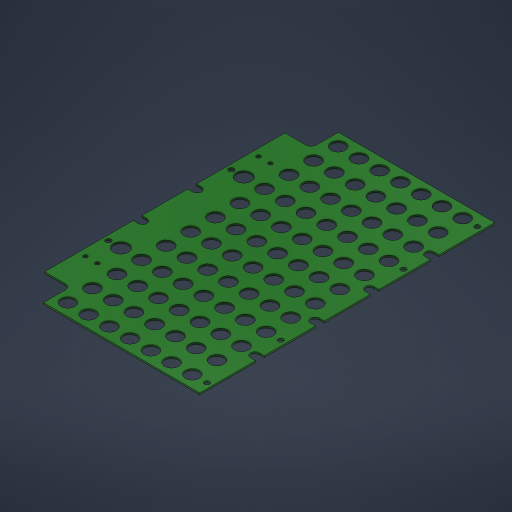
# Autodesk Inventor part: PCB
Saved by Autodesk Inventor 2023.5 (Build 275446000, 446)
## iProperties
Created: 2025-03-26
Part Number: PCB
Material: PC/ABS-Kunststoff
Document SubType Name: Modeling
Designer: David Lill
Density: 0.357273 g/cm^3
Appearance: Glatt - Waldgrün
Author: David Lill
Autodesk Inventor part; units mm, degrees
ref_plane "YZ Plane" through (0, 0, 0) normal (1, 0, 0) x (0, 1, 0)
ref_plane "XZ Plane" through (0, 0, 0) normal (0, 1, 0) x (-1, 0, 0)
ref_plane "XY Plane" through (0, 0, 0) normal (0, 0, 1) x (1, 0, 0)
sketch "Skizze1" plane through (0, 0, 0) normal (0, 0, 1) x (1, 0, 0)
  arc A0 (0, 11.25) -> (-14.9586, 20.25) centre (-14.9586, 3.3189) ccw
  arc A1 (-14.9586, 2.25) -> (-14.9586, 20.25) centre (-18, 11.25) ccw
  arc A2 (-14.9586, 2.25) -> (0, 11.25) centre (-14.9586, 19.1811) ccw
  arc A3 (0, 78.75) -> (-14.9586, 87.75) centre (-14.9586, 70.8189) ccw
  arc A4 (-14.9586, 69.75) -> (-14.9586, 87.75) centre (-18, 78.75) ccw
  arc A5 (-14.9586, 69.75) -> (0, 78.75) centre (-14.9586, 86.6811) ccw
  line L0 (0, 0) -> (0, 270)
  arc A6 (-4.65, 164) -> (-4.65, 156) centre (-4.65, 160) ccw
  line L1 (-4.65, 156) -> (0, 156)
  line L2 (0, 0) -> (0, 270)
  arc A7 (-4.65, 219) -> (-4.65, 211) centre (-4.65, 215) ccw
  line L3 (-4.65, 211) -> (0, 211)
  line L4 (0, 135) -> (-167, 135)
  line L5 (0, 270) -> (-167, 270)
  line L6 (-167, 270) -> (-167, 0)
  line L7 (-167, 270) -> (-167, 0)
  line L8 (-167, 0) -> (0, 0)
  line L9 (0, 0) -> (-167, 0)
  line L10 (-144.5, 31.5) -> (-165.5, 31.5)
  line L11 (-165.5, 31.5) -> (-165.5, 58.5)
  line L12 (-165.5, 58.5) -> (-144.5, 58.5)
  line L13 (-144.5, 58.5) -> (-144.5, 31.5)
  line L14 (-144.5, 238.5) -> (-165.5, 238.5)
  line L15 (-165.5, 238.5) -> (-165.5, 211.5)
  line L16 (-165.5, 211.5) -> (-144.5, 211.5)
  line L17 (-144.5, 211.5) -> (-144.5, 238.5)
  arc A8 (0, 258.75) -> (-14.9586, 267.75) centre (-14.9586, 250.8189) ccw
  arc A9 (-14.9586, 249.75) -> (0, 258.75) centre (-14.9586, 266.6811) ccw
  arc A10 (-14.9586, 249.75) -> (-14.9586, 267.75) centre (-18, 258.75) ccw
  arc A11 (0, 191.25) -> (-14.9586, 200.25) centre (-14.9586, 183.3189) ccw
  arc A12 (-14.9586, 182.25) -> (-14.9586, 200.25) centre (-18, 191.25) ccw
  arc A13 (-14.9586, 182.25) -> (0, 191.25) centre (-14.9586, 199.1811) ccw
  line L18 (-135.0414, 87.75) -> (-158, 87.75)
  arc A14 (-158, 87.75) -> (-158, 69.75) centre (-158, 78.75) ccw
  line L19 (-158, 69.75) -> (-135.0414, 69.75)
  arc A15 (-135.0414, 87.75) -> (-135.0414, 69.75) centre (-132, 78.75) ccw
  line L20 (-158, 182.25) -> (-135.0414, 182.25)
  arc A16 (-135.0414, 200.25) -> (-135.0414, 182.25) centre (-132, 191.25) ccw
  line L21 (-135.0414, 200.25) -> (-158, 200.25)
  arc A17 (-158, 200.25) -> (-158, 182.25) centre (-158, 191.25) ccw
  line L22 (-143, 0) -> (-143, 55)
  arc A18 (-143, 55) -> (-148, 60) centre (-148, 55) ccw
  line L23 (-148, 60) -> (-167, 60)
  line L24 (-167, 25) -> (-148, 25)
  arc A19 (-143, 20) -> (-148, 25) centre (-148, 20) ccw
  line L25 (-143, 270) -> (-143, 215)
  arc A20 (-148, 210) -> (-143, 215) centre (-148, 215) ccw
  line L26 (-148, 210) -> (-167, 210)
  line L27 (-167, 245) -> (-148, 245)
  arc A21 (-148, 245) -> (-143, 250) centre (-148, 250) ccw
  line L28 (0, 219) -> (-4.65, 219)
  arc A22 (-4.65, 219) -> (-4.65, 211) centre (-4.65, 215) ccw
  line L29 (-4.65, 211) -> (0, 211)
  line L30 (0, 164) -> (-4.65, 164)
  arc A23 (-4.65, 164) -> (-4.65, 156) centre (-4.65, 160) ccw
  line L31 (-4.65, 156) -> (0, 156)
  line L32 (-167, 156) -> (-162.35, 156)
  arc A24 (-162.35, 156) -> (-162.35, 164) centre (-162.35, 160) ccw
  line L33 (-162.35, 164) -> (-167, 164)
  line L34 (0, 59) -> (-4.65, 59)
  arc A25 (-4.65, 59) -> (-4.65, 51) centre (-4.65, 55) ccw
  line L35 (-4.65, 51) -> (0, 51)
  line L36 (0, 106) -> (-4.65, 106)
  arc A26 (-4.65, 114) -> (-4.65, 106) centre (-4.65, 110) ccw
  line L37 (-4.65, 114) -> (0, 114)
  line L38 (-167, 106) -> (-162.35, 106)
  arc A27 (-162.35, 106) -> (-162.35, 114) centre (-162.35, 110) ccw
  line L39 (-162.35, 114) -> (-167, 114)
  circle A28 centre (-18, 236.25) radius 9
  circle A29 centre (-18, 258.75) radius 9
  circle A30 centre (-18, 213.75) radius 9
  circle A31 centre (-18, 168.75) radius 9
  circle A32 centre (-18, 123.75) radius 9
  circle A33 centre (-18, 78.75) radius 9
  circle A34 centre (-18, 33.75) radius 9
  circle A35 centre (-18, 11.25) radius 9
  circle A36 centre (-18, 56.25) radius 9
  circle A37 centre (-18, 101.25) radius 9
  circle A38 centre (-18, 146.25) radius 9
  circle A39 centre (-18, 191.25) radius 9
  circle A40 centre (-37, 236.25) radius 9
  circle A41 centre (-37, 258.75) radius 9
  circle A42 centre (-37, 213.75) radius 9
  circle A43 centre (-37, 168.75) radius 9
  circle A44 centre (-37, 123.75) radius 9
  circle A45 centre (-37, 78.75) radius 9
  circle A46 centre (-37, 33.75) radius 9
  circle A47 centre (-37, 11.25) radius 9
  circle A48 centre (-37, 56.25) radius 9
  circle A49 centre (-37, 101.25) radius 9
  circle A50 centre (-37, 146.25) radius 9
  circle A51 centre (-37, 191.25) radius 9
  circle A52 centre (-56, 236.25) radius 9
  circle A53 centre (-56, 258.75) radius 9
  circle A54 centre (-56, 213.75) radius 9
  circle A55 centre (-56, 168.75) radius 9
  circle A56 centre (-56, 123.75) radius 9
  circle A57 centre (-56, 78.75) radius 9
  circle A58 centre (-56, 33.75) radius 9
  circle A59 centre (-56, 11.25) radius 9
  circle A60 centre (-56, 56.25) radius 9
  circle A61 centre (-56, 101.25) radius 9
  circle A62 centre (-56, 146.25) radius 9
  circle A63 centre (-56, 191.25) radius 9
  circle A64 centre (-75, 236.25) radius 9
  circle A65 centre (-75, 258.75) radius 9
  circle A66 centre (-75, 213.75) radius 9
  circle A67 centre (-75, 168.75) radius 9
  circle A68 centre (-75, 123.75) radius 9
  circle A69 centre (-75, 78.75) radius 9
  circle A70 centre (-75, 33.75) radius 9
  circle A71 centre (-75, 11.25) radius 9
  circle A72 centre (-75, 56.25) radius 9
  circle A73 centre (-75, 101.25) radius 9
  circle A74 centre (-75, 146.25) radius 9
  circle A75 centre (-75, 191.25) radius 9
  circle A76 centre (-94, 236.25) radius 9
  circle A77 centre (-94, 258.75) radius 9
  circle A78 centre (-94, 213.75) radius 9
  circle A79 centre (-94, 168.75) radius 9
  circle A80 centre (-94, 123.75) radius 9
  circle A81 centre (-94, 78.75) radius 9
  circle A82 centre (-94, 33.75) radius 9
  circle A83 centre (-94, 11.25) radius 9
  circle A84 centre (-94, 56.25) radius 9
  circle A85 centre (-94, 101.25) radius 9
  circle A86 centre (-94, 146.25) radius 9
  circle A87 centre (-94, 191.25) radius 9
  circle A88 centre (-113, 236.25) radius 9
  circle A89 centre (-113, 258.75) radius 9
  circle A90 centre (-113, 213.75) radius 9
  circle A91 centre (-113, 168.75) radius 9
  circle A92 centre (-113, 123.75) radius 9
  circle A93 centre (-113, 78.75) radius 9
  circle A94 centre (-113, 33.75) radius 9
  circle A95 centre (-113, 11.25) radius 9
  circle A96 centre (-113, 56.25) radius 9
  circle A97 centre (-113, 101.25) radius 9
  circle A98 centre (-113, 146.25) radius 9
  circle A99 centre (-113, 191.25) radius 9
  circle A100 centre (-132, 236.25) radius 9
  circle A101 centre (-132, 191.25) radius 9
  circle A102 centre (-132, 146.25) radius 9
  circle A103 centre (-132, 101.25) radius 9
  circle A104 centre (-132, 56.25) radius 9
  circle A105 centre (-132, 11.25) radius 9
  circle A106 centre (-132, 33.75) radius 9
  circle A107 centre (-132, 78.75) radius 9
  circle A108 centre (-132, 123.75) radius 9
  circle A109 centre (-132, 168.75) radius 9
  circle A110 centre (-132, 213.75) radius 9
  circle A111 centre (-132, 258.75) radius 9
  line L40 (0, 0) -> (0, 270)
  line L41 (-167, 0) -> (0, 0)
  line L42 (-167, 270) -> (-167, 0)
  line L43 (-167, 0) -> (0, 0)
  line L44 (0, 270) -> (-167, 270)
  line L45 (0, 135) -> (-167, 135)
  line L46 (-14.9586, 2.25) -> (-18, 2.25)
  circle A112 centre (-18, 11.25) radius 9
  circle A113 centre (-4.65, 11.25) radius 2.5
  circle A114 centre (-4.65, 78.75) radius 2.5
  circle A115 centre (-4.65, 191.25) radius 2.5
  circle A116 centre (-4.65, 258.75) radius 2.5
  circle A117 centre (-162.35, 78.75) radius 2.5
  circle A118 centre (-162.35, 191.25) radius 2.5
  circle A119 centre (-151, 78.75) radius 7
  circle A120 centre (-151, 191.25) radius 7
  circle A121 centre (-160.45, 55.8) radius 1.95
  circle A122 centre (-149.55, 55.8) radius 1.95
  circle A123 centre (-160.45, 214.2) radius 1.95
  circle A124 centre (-149.55, 214.2) radius 1.95
  circle A125 centre (-132, 11.25) radius 6.5
  circle A126 centre (-113, 11.25) radius 6.5
  circle A127 centre (-94, 11.25) radius 6.5
  circle A128 centre (-75, 11.25) radius 6.5
  circle A129 centre (-56, 11.25) radius 6.5
  circle A130 centre (-37, 11.25) radius 6.5
  circle A131 centre (-18, 11.25) radius 6.5
  circle A132 centre (-132, 33.75) radius 6.5
  circle A133 centre (-113, 33.75) radius 6.5
  circle A134 centre (-94, 33.75) radius 6.5
  circle A135 centre (-75, 33.75) radius 6.5
  circle A136 centre (-56, 33.75) radius 6.5
  circle A137 centre (-37, 33.75) radius 6.5
  circle A138 centre (-18, 33.75) radius 6.5
  circle A139 centre (-132, 56.25) radius 6.5
  circle A140 centre (-113, 56.25) radius 6.5
  circle A141 centre (-94, 56.25) radius 6.5
  circle A142 centre (-75, 56.25) radius 6.5
  circle A143 centre (-56, 56.25) radius 6.5
  circle A144 centre (-37, 56.25) radius 6.5
  circle A145 centre (-18, 56.25) radius 6.5
  circle A146 centre (-132, 78.75) radius 6.5
  circle A147 centre (-113, 78.75) radius 6.5
  circle A148 centre (-94, 78.75) radius 6.5
  circle A149 centre (-75, 78.75) radius 6.5
  circle A150 centre (-56, 78.75) radius 6.5
  circle A151 centre (-37, 78.75) radius 6.5
  circle A152 centre (-18, 78.75) radius 6.5
  circle A153 centre (-132, 101.25) radius 6.5
  circle A154 centre (-113, 101.25) radius 6.5
  circle A155 centre (-94, 101.25) radius 6.5
  circle A156 centre (-75, 101.25) radius 6.5
  circle A157 centre (-56, 101.25) radius 6.5
  circle A158 centre (-37, 101.25) radius 6.5
  circle A159 centre (-18, 101.25) radius 6.5
  circle A160 centre (-132, 123.75) radius 6.5
  circle A161 centre (-113, 123.75) radius 6.5
  circle A162 centre (-94, 123.75) radius 6.5
  circle A163 centre (-75, 123.75) radius 6.5
  circle A164 centre (-56, 123.75) radius 6.5
  circle A165 centre (-37, 123.75) radius 6.5
  circle A166 centre (-18, 123.75) radius 6.5
  circle A167 centre (-132, 146.25) radius 6.5
  circle A168 centre (-113, 146.25) radius 6.5
  circle A169 centre (-94, 146.25) radius 6.5
  circle A170 centre (-75, 146.25) radius 6.5
  circle A171 centre (-56, 146.25) radius 6.5
  circle A172 centre (-37, 146.25) radius 6.5
  circle A173 centre (-18, 146.25) radius 6.5
  circle A174 centre (-132, 168.75) radius 6.5
  circle A175 centre (-113, 168.75) radius 6.5
  circle A176 centre (-94, 168.75) radius 6.5
  circle A177 centre (-75, 168.75) radius 6.5
  circle A178 centre (-56, 168.75) radius 6.5
  circle A179 centre (-37, 168.75) radius 6.5
  circle A180 centre (-18, 168.75) radius 6.5
  circle A181 centre (-132, 191.25) radius 6.5
  circle A182 centre (-113, 191.25) radius 6.5
  circle A183 centre (-94, 191.25) radius 6.5
  circle A184 centre (-75, 191.25) radius 6.5
  circle A185 centre (-56, 191.25) radius 6.5
  circle A186 centre (-37, 191.25) radius 6.5
  circle A187 centre (-18, 191.25) radius 6.5
  circle A188 centre (-132, 213.75) radius 6.5
  circle A189 centre (-113, 213.75) radius 6.5
  circle A190 centre (-94, 213.75) radius 6.5
  circle A191 centre (-75, 213.75) radius 6.5
  circle A192 centre (-56, 213.75) radius 6.5
  circle A193 centre (-37, 213.75) radius 6.5
  circle A194 centre (-18, 213.75) radius 6.5
  circle A195 centre (-132, 236.25) radius 6.5
  circle A196 centre (-113, 236.25) radius 6.5
  circle A197 centre (-94, 236.25) radius 6.5
  circle A198 centre (-75, 236.25) radius 6.5
  circle A199 centre (-56, 236.25) radius 6.5
  circle A200 centre (-37, 236.25) radius 6.5
  circle A201 centre (-18, 236.25) radius 6.5
  circle A202 centre (-132, 258.75) radius 6.5
  circle A203 centre (-113, 258.75) radius 6.5
  circle A204 centre (-94, 258.75) radius 6.5
  circle A205 centre (-75, 258.75) radius 6.5
  circle A206 centre (-56, 258.75) radius 6.5
  circle A207 centre (-37, 258.75) radius 6.5
  circle A208 centre (-18, 258.75) radius 6.5
  point P0 (-155, 58.5)
  point P1 (0, 114)
  point P2 (0, 156)
  point P3 (-4.65, 156)
  point P4 (-4.65, 164)
  point P5 (0, 211)
  point P6 (-4.65, 211)
  point P7 (-143, 250)
  dimension "d8" = 10.9
  dimension "d9" = 5.45
  dimension "d10" = 2.7
  dimension "d11" = 3.9
  dimension "d12" = 13
  dimension "d15" = 19
  dimension "d18" = 22.5
  constraints: 209 centre point, 94 end point, 56 point on circle, 36 horizontal, 13 vertical, 2 symmetric about line, 1 coincident, 1 equal radius, 1 horizontal alignment, 1 midpoint, 560 other
  measures "d8" distance of A122.centre A121.centre
  measures "d9" horizontal distance of point (-155, 58.5) A121.centre
  measures "d10" distance from line of L12 A121.centre
  measures "d11" diameter of A121
  measures "d12" diameter of A125
  measures "d15" distance of A125.centre A126.centre
  measures "d18" distance of A125.centre A132.centre
extrude "Extrusion1" add sketch "Skizze1" along normal blind 1.6 contours A2 A1 A0 | A5 A4 A3 | A14 L18 A15 L19 | L0 L8 L22 A18 L23 L6 L38 A27 L39 L4 L37 A26 L36 L34 A25 L35 | A19 L24 L6 L23 A18 L22 | A13 A12 A11 | A9 A10 A8 | A17 L21 A16 L20 | L4 L6 L32 A24 L33 L26 A20 L25 L5 L0 L28 A7 L3 L30 A6 L1 | L6 L27 A21 L25 A20 L26 | L10 L11 L12 L13 | L17 L16 L15 L14 | A28 | A29 | A30 | A31 | A32 | A33 | A34 | A35 | A36 | A37 | A38 | A39 | A40 | A41 | A42 | A43 | A44 | A45 | A46 | A47 | A48 | A49 | A50 | A51 | A52 | A53 | A54 | A55 | A56 | A57 | A58 | A59 | A60 | A61 | A62 | A63 | A64 | A65 | A66 | A67 | A68 | A69 | A70 | A71 | A72 | A73 | A74 | A75 | A76 | A77 | A78 | A79 | A80 | A81 | A82 | A83 | A84 | A85 | A86 | A87 | A88 | A89 | A90 | A91 | A92 | A93 | A94 | A95 | A96 | A97 | A98 | A99 | A100 | A101 | A102 | A103 | A104 | A105 | A106 | A107 | A108 | A109 | A110 | A111
equation "\"d9\" = 0.5 * d8"
